Autodesk Inventor part; units mm, degrees
(part 2 of 2)
  spline S170 degree 2 poles (-5.6708, -24.2315) (-5.4763, -24.2315) (-5.2794, -24.0127) (-5.2794, -23.8036) knots 0 0 0 1 2 2 2
  spline S171 degree 2 poles (-5.2794, -23.8036) (-5.2794, -23.6261) (-5.4326, -23.3344) (-5.5468, -23.208) knots 0 0 0 1 2 2 2
  spline S172 degree 2 poles (-4.9925, -22.8773) (-4.9196, -22.9649) (-4.7032, -23.0961) (-4.6084, -23.0961) knots 0 0 0 1 2 2 2
  spline S173 degree 2 poles (-4.6084, -23.0961) (-4.5428, -23.0961) (-4.4601, -23.0208) (-4.4601, -22.9454) knots 0 0 0 1 2 2 2
  spline S174 degree 2 poles (-4.4601, -22.9454) (-4.4601, -22.9041) (-4.4796, -22.8287) (-4.4893, -22.8044) knots 0 0 0 1 2 2 2
  line L358 (-4.4893, -22.8044) -> (-4.4893, -22.7825)
  line L359 (-4.4893, -22.7825) -> (-4.2073, -22.7825)
  spline S175 degree 2 poles (-4.2073, -22.7825) (-4.183, -22.8409) (-4.1611, -22.9697) (-4.1611, -23.0232) knots 0 0 0 1 2 2 2
  spline S176 degree 2 poles (-4.1611, -23.0232) (-4.1611, -23.2031) (-4.3483, -23.4073) (-4.516, -23.4073) knots 0 0 0 1 2 2 2
  spline S177 degree 2 poles (-4.516, -23.4073) (-4.6473, -23.4073) (-4.9074, -23.2663) (-4.9925, -23.1764) knots 0 0 0 1 2 2 2
  line L360 (-4.9925, -23.1764) -> (-4.9925, -22.8773)
  spline S178 degree 2 poles (-4.9488, -21.6156) (-4.9488, -21.9243) (-5.3013, -22.272) (-5.683, -22.272) knots 0 0 0 1 2 2 2
  line L361 (-5.683, -22.272) -> (-6.9301, -22.272)
  line L362 (-6.9301, -22.272) -> (-6.9301, -22.5273)
  line L363 (-6.9301, -22.5273) -> (-7.2438, -22.5273)
  line L364 (-7.2438, -22.5273) -> (-7.2438, -22.272)
  line L365 (-7.2438, -22.272) -> (-7.8904, -22.272)
  line L366 (-7.8904, -22.272) -> (-7.8904, -21.8927)
  line L367 (-7.8904, -21.8927) -> (-7.2438, -21.8927)
  line L368 (-7.2438, -21.8927) -> (-7.2438, -21.195)
  line L369 (-7.2438, -21.195) -> (-6.9301, -21.195)
  line L370 (-6.9301, -21.195) -> (-6.9301, -21.8927)
  line L371 (-6.9301, -21.8927) -> (-5.858, -21.8927)
  spline S179 degree 2 poles (-5.858, -21.8927) (-5.6878, -21.8927) (-5.5006, -21.8806) (-5.4204, -21.8393) knots 0 0 0 1 2 2 2
  spline S180 degree 2 poles (-5.4204, -21.8393) (-5.3499, -21.8052) (-5.2794, -21.6521) (-5.2794, -21.5208) knots 0 0 0 1 2 2 2
  spline S181 degree 2 poles (-5.2794, -21.5208) (-5.2794, -21.4284) (-5.3353, -21.2558) (-5.3523, -21.2169) knots 0 0 0 1 2 2 2
  line L372 (-5.3523, -21.2169) -> (-5.3523, -21.195)
  line L373 (-5.3523, -21.195) -> (-5.012, -21.195)
  spline S182 degree 2 poles (-5.012, -21.195) (-4.9828, -21.302) (-4.9488, -21.5208) (-4.9488, -21.6156) knots 0 0 0 1 2 2 2
  line L374 (-7.2438, -19.148) -> (-4.1635, -20.3587)
  line L375 (-4.1635, -20.3587) -> (-4.1635, -20.7647)
  line L376 (-4.1635, -20.7647) -> (-5.1019, -20.3611)
  line L377 (-5.1019, -20.3611) -> (-7.2438, -21.178)
  line L378 (-7.2438, -21.178) -> (-7.2438, -20.7696)
  line L379 (-7.2438, -20.7696) -> (-5.576, -20.1545)
  line L380 (-5.576, -20.1545) -> (-7.2438, -19.5418)
  line L381 (-7.2438, -19.5418) -> (-7.2438, -19.148)
  line L382 (-5.1301, -41.1451) -> (-5.1301, -41.6022)
  line L383 (-5.1301, -41.6022) -> (-6.3262, -42.3315)
  line L384 (-6.3262, -42.3315) -> (-5.1301, -43.0754)
  line L385 (-5.1301, -43.0754) -> (-5.1301, -43.5057)
  line L386 (-5.1301, -43.5057) -> (-6.6325, -42.5503)
  line L387 (-6.6325, -42.5503) -> (-8.1301, -43.4765)
  line L388 (-8.1301, -43.4765) -> (-8.1301, -43.0195)
  line L389 (-8.1301, -43.0195) -> (-6.9558, -42.3047)
  line L390 (-6.9558, -42.3047) -> (-8.1301, -41.5754)
  line L391 (-8.1301, -41.5754) -> (-8.1301, -41.1451)
  line L392 (-8.1301, -41.1451) -> (-6.652, -42.0835)
  line L393 (-6.652, -42.0835) -> (-5.1301, -41.1451)
  line L394 (-8.1301, -38.7237) -> (-6.4575, -39.7375)
  line L395 (-6.4575, -39.7375) -> (-5.1301, -39.7375)
  line L396 (-5.1301, -39.7375) -> (-5.1301, -40.1362)
  line L397 (-5.1301, -40.1362) -> (-6.4161, -40.1362)
  line L398 (-6.4161, -40.1362) -> (-8.1301, -41.15)
  line L399 (-8.1301, -41.15) -> (-8.1301, -40.7075)
  line L400 (-8.1301, -40.7075) -> (-6.81, -39.9344)
  line L401 (-6.81, -39.9344) -> (-8.1301, -39.1467)
  line L402 (-8.1301, -39.1467) -> (-8.1301, -38.7237)
  line L403 (-5.1301, -36.5333) -> (-5.1301, -38.6289)
  line L404 (-5.1301, -38.6289) -> (-5.502, -38.6289)
  line L405 (-5.502, -38.6289) -> (-7.7751, -37.0244)
  line L406 (-7.7751, -37.0244) -> (-7.7751, -38.556)
  line L407 (-7.7751, -38.556) -> (-8.1301, -38.556)
  line L408 (-8.1301, -38.556) -> (-8.1301, -36.5746)
  line L409 (-8.1301, -36.5746) -> (-7.7703, -36.5746)
  line L410 (-7.7703, -36.5746) -> (-5.485, -38.1962)
  line L411 (-5.485, -38.1962) -> (-5.485, -36.5333)
  line L412 (-5.485, -36.5333) -> (-5.1301, -36.5333)
  spline S183 degree 2 poles (4.3705, -37.8576) (4.565, -37.8576) (4.9151, -37.9962) (5.0366, -38.1201) knots 0 0 0 1 2 2 2
  spline S184 degree 2 poles (5.0366, -38.1201) (5.1898, -38.2757) (5.3478, -38.6963) (5.3478, -39.0172) knots 0 0 0 1 2 2 2
  line L413 (5.3478, -39.0172) -> (5.3478, -39.3552)
  line L414 (5.3478, -39.3552) -> (6.4661, -39.3552)
  line L415 (6.4661, -39.3552) -> (6.4661, -39.7539)
  line L416 (6.4661, -39.7539) -> (3.4661, -39.7539)
  line L417 (3.4661, -39.7539) -> (3.4661, -39.0002)
  spline S185 degree 2 poles (3.4661, -39.0002) (3.4661, -38.7328) (3.5536, -38.3584) (3.6533, -38.215) knots 0 0 0 1 2 2 2
  spline S186 degree 2 poles (3.6533, -38.215) (3.7676, -38.0472) (4.1201, -37.8576) (4.3705, -37.8576) knots 0 0 0 1 2 2 2
  spline S187 degree 2 poles (4.3827, -38.2733) (4.2271, -38.2733) (3.9985, -38.3803) (3.9256, -38.4897) knots 0 0 0 1 2 2 2
  spline S188 degree 2 poles (3.9256, -38.4897) (3.8624, -38.5845) (3.8113, -38.8373) (3.8113, -39.0245) knots 0 0 0 1 2 2 2
  line L418 (3.8113, -39.0245) -> (3.8113, -39.3552)
  line L419 (3.8113, -39.3552) -> (5.0075, -39.3552)
  line L420 (5.0075, -39.3552) -> (5.0075, -39.0829)
  spline S189 degree 2 poles (5.0075, -39.0829) (5.0075, -38.8398) (4.9297, -38.5407) (4.8275, -38.4435) knots 0 0 0 1 2 2 2
  spline S190 degree 2 poles (4.8275, -38.4435) (4.7376, -38.3535) (4.5261, -38.2733) (4.3827, -38.2733) knots 0 0 0 1 2 2 2
  line L421 (4.6209, -36.3138) -> (4.6209, -36.3333)
  spline S191 degree 2 poles (4.6209, -36.3333) (4.6087, -36.377) (4.6039, -36.4719) (4.6039, -36.5375) knots 0 0 0 1 2 2 2
  spline S192 degree 2 poles (4.6039, -36.5375) (4.6039, -36.6907) (4.7376, -36.9921) (4.8689, -37.1283) knots 0 0 0 1 2 2 2
  line L422 (4.8689, -37.1283) -> (6.4661, -37.1283)
  line L423 (6.4661, -37.1283) -> (6.4661, -37.5075)
  line L424 (6.4661, -37.5075) -> (4.2149, -37.5075)
  line L425 (4.2149, -37.5075) -> (4.2149, -37.1283)
  line L426 (4.2149, -37.1283) -> (4.5504, -37.1283)
  spline S193 degree 2 poles (4.5504, -37.1283) (4.3656, -36.9216) (4.2149, -36.6129) (4.2149, -36.467) knots 0 0 0 1 2 2 2
  spline S194 degree 2 poles (4.2149, -36.467) (4.2149, -36.4086) (4.2198, -36.3503) (4.2271, -36.3138) knots 0 0 0 1 2 2 2
  line L427 (4.2271, -36.3138) -> (4.6209, -36.3138)
  line L428 (6.4661, -34.5415) -> (6.4661, -36.1947)
  line L429 (6.4661, -36.1947) -> (6.1841, -36.1947)
  line L430 (6.1841, -36.1947) -> (4.5261, -35.018)
  line L431 (4.5261, -35.018) -> (4.5261, -36.1461)
  line L432 (4.5261, -36.1461) -> (4.2149, -36.1461)
  line L433 (4.2149, -36.1461) -> (4.2149, -34.5634)
  line L434 (4.2149, -34.5634) -> (4.4848, -34.5634)
  line L435 (4.4848, -34.5634) -> (6.1476, -35.7449)
  line L436 (6.1476, -35.7449) -> (6.1476, -34.5415)
  line L437 (6.1476, -34.5415) -> (6.4661, -34.5415)
  spline S195 degree 2 poles (6.5172, -33.2093) (6.5172, -33.749) (5.9118, -34.3422) (5.3527, -34.3422) knots 0 0 0 1 2 2 2
  spline S196 degree 2 poles (5.3527, -34.3422) (4.8032, -34.3422) (4.1517, -33.766) (4.1517, -33.3017) knots 0 0 0 1 2 2 2
  spline S197 degree 2 poles (4.1517, -33.3017) (4.1517, -33.0926) (4.2733, -32.7693) (4.4021, -32.6501) knots 0 0 0 1 2 2 2
  spline S198 degree 2 poles (4.4021, -32.6501) (4.531, -32.5286) (4.9029, -32.3997) (5.1728, -32.3997) knots 0 0 0 1 2 2 2
  line L438 (5.1728, -32.3997) -> (5.3794, -32.3997)
  line L439 (5.3794, -32.3997) -> (5.3794, -33.9581)
  spline S199 degree 2 poles (5.3794, -33.9581) (5.7708, -33.9581) (6.1865, -33.5642) (6.1865, -33.2142) knots 0 0 0 1 2 2 2
  spline S200 degree 2 poles (6.1865, -33.2142) (6.1865, -33.0902) (6.1306, -32.8495) (6.0869, -32.7522) knots 0 0 0 1 2 2 2
  spline S201 degree 2 poles (6.0869, -32.7522) (6.0382, -32.6501) (5.9532, -32.5091) (5.9143, -32.4629) knots 0 0 0 1 2 2 2
  line L440 (5.9143, -32.4629) -> (5.9143, -32.4411)
  line L441 (5.9143, -32.4411) -> (6.3275, -32.4411)
  spline S202 degree 2 poles (6.3275, -32.4411) (6.3543, -32.5067) (6.4321, -32.706) (6.454, -32.7838) knots 0 0 0 1 2 2 2
  spline S203 degree 2 poles (6.454, -32.7838) (6.4856, -32.8932) (6.5172, -33.0731) (6.5172, -33.2093) knots 0 0 0 1 2 2 2
  spline S204 degree 2 poles (5.0901, -32.7693) (4.9369, -32.7741) (4.7133, -32.8373) (4.6379, -32.8981) knots 0 0 0 1 2 2 2
  spline S205 degree 2 poles (4.6379, -32.8981) (4.5528, -32.9637) (4.4629, -33.1704) (4.4629, -33.3236) knots 0 0 0 1 2 2 2
  spline S206 degree 2 poles (4.4629, -33.3236) (4.4629, -33.4743) (4.5528, -33.6858) (4.6404, -33.7733) knots 0 0 0 1 2 2 2
  spline S207 degree 2 poles (4.6404, -33.7733) (4.7303, -33.8584) (4.9467, -33.9459) (5.0901, -33.9581) knots 0 0 0 1 2 2 2
  line L442 (5.0901, -33.9581) -> (5.0901, -32.7693)
  spline S208 degree 2 poles (6.8259, -31.9354) (6.8429, -31.8965) (6.8964, -31.7482) (6.9183, -31.6534) knots 0 0 0 1 2 2 2
  spline S209 degree 2 poles (6.9183, -31.6534) (6.9451, -31.5488) (6.9767, -31.3714) (6.9767, -31.2668) knots 0 0 0 1 2 2 2
  spline S210 degree 2 poles (6.9767, -31.2668) (6.9767, -31.0918) (6.8843, -30.8487) (6.8016, -30.7806) knots 0 0 0 1 2 2 2
  spline S211 degree 2 poles (6.8016, -30.7806) (6.719, -30.715) (6.5026, -30.6639) (6.364, -30.6639) knots 0 0 0 1 2 2 2
  line L443 (6.364, -30.6639) -> (6.1671, -30.6639)
  spline S212 degree 2 poles (6.1671, -30.6639) (6.3008, -30.8171) (6.4272, -31.1112) (6.4272, -31.3325) knots 0 0 0 1 2 2 2
  spline S213 degree 2 poles (6.4272, -31.3325) (6.4272, -31.7166) (5.8559, -32.1712) (5.3186, -32.1712) knots 0 0 0 1 2 2 2
  spline S214 degree 2 poles (5.3186, -32.1712) (5.0391, -32.1712) (4.6063, -32.0132) (4.4532, -31.8819) knots 0 0 0 1 2 2 2
  spline S215 degree 2 poles (4.4532, -31.8819) (4.3097, -31.7555) (4.1517, -31.4078) (4.1517, -31.2231) knots 0 0 0 1 2 2 2
  spline S216 degree 2 poles (4.1517, -31.2231) (4.1517, -31.048) (4.2344, -30.7928) (4.3097, -30.6639) knots 0 0 0 1 2 2 2
  line L444 (4.3097, -30.6639) -> (4.2149, -30.642)
  line L445 (4.2149, -30.642) -> (4.2149, -30.2847)
  line L446 (4.2149, -30.2847) -> (6.2084, -30.2847)
  spline S217 degree 2 poles (6.2084, -30.2847) (6.7822, -30.2847) (7.317, -30.783) (7.317, -31.296) knots 0 0 0 1 2 2 2
  spline S218 degree 2 poles (7.317, -31.296) (7.317, -31.4613) (7.2635, -31.8065) (7.2198, -31.9548) knots 0 0 0 1 2 2 2
  line L447 (7.2198, -31.9548) -> (6.8259, -31.9548)
  line L448 (6.8259, -31.9548) -> (6.8259, -31.9354)
  line L449 (5.8559, -30.6639) -> (4.6185, -30.6639)
  spline S219 degree 2 poles (4.6185, -30.6639) (4.5504, -30.8049) (4.4921, -31.0432) (4.4921, -31.1623) knots 0 0 0 1 2 2 2
  spline S220 degree 2 poles (4.4921, -31.1623) (4.4921, -31.4492) (4.9151, -31.7798) (5.3113, -31.7798) knots 0 0 0 1 2 2 2
  spline S221 degree 2 poles (5.3113, -31.7798) (5.6857, -31.7798) (6.0771, -31.5294) (6.0771, -31.2474) knots 0 0 0 1 2 2 2
  spline S222 degree 2 poles (6.0771, -31.2474) (6.0771, -31.0991) (5.9605, -30.7879) (5.8559, -30.6639) knots 0 0 0 1 2 2 2
  line L450 (6.4661, -27.9848) -> (6.4661, -28.3641)
  line L451 (6.4661, -28.3641) -> (6.2181, -28.3641)
  spline S223 degree 2 poles (6.2181, -28.3641) (6.3713, -28.5391) (6.5293, -28.8527) (6.5293, -29.0472) knots 0 0 0 1 2 2 2
  spline S224 degree 2 poles (6.5293, -29.0472) (6.5293, -29.1931) (6.4321, -29.4532) (6.3275, -29.548) knots 0 0 0 1 2 2 2
  spline S225 degree 2 poles (6.3275, -29.548) (6.223, -29.6453) (5.9045, -29.7522) (5.676, -29.7522) knots 0 0 0 1 2 2 2
  line L452 (5.676, -29.7522) -> (4.2149, -29.7522)
  line L453 (4.2149, -29.7522) -> (4.2149, -29.373)
  line L454 (4.2149, -29.373) -> (5.4985, -29.373)
  spline S226 degree 2 poles (5.4985, -29.373) (5.6784, -29.373) (5.9143, -29.3462) (6.0018, -29.3001) knots 0 0 0 1 2 2 2
  spline S227 degree 2 poles (6.0018, -29.3001) (6.0893, -29.2539) (6.1695, -29.0958) (6.1695, -28.9475) knots 0 0 0 1 2 2 2
  spline S228 degree 2 poles (6.1695, -28.9475) (6.1695, -28.809) (6.0115, -28.4954) (5.8972, -28.3641) knots 0 0 0 1 2 2 2
  line L455 (5.8972, -28.3641) -> (4.2149, -28.3641)
  line L456 (4.2149, -28.3641) -> (4.2149, -27.9848)
  line L457 (4.2149, -27.9848) -> (6.4661, -27.9848)
  spline S229 degree 2 poles (5.304, -25.5488) (5.8559, -25.5488) (6.5293, -26.0837) (6.5293, -26.4872) knots 0 0 0 1 2 2 2
  spline S230 degree 2 poles (6.5293, -26.4872) (6.5293, -26.6696) (6.4394, -26.9297) (6.3616, -27.0561) knots 0 0 0 1 2 2 2
  line L458 (6.3616, -27.0561) -> (6.4661, -27.0804)
  line L459 (6.4661, -27.0804) -> (6.4661, -27.4354)
  line L460 (6.4661, -27.4354) -> (3.3324, -27.4354)
  line L461 (3.3324, -27.4354) -> (3.3324, -27.0561)
  line L462 (3.3324, -27.0561) -> (4.4507, -27.0561)
  spline S231 degree 2 poles (4.4507, -27.0561) (4.3219, -26.9127) (4.1517, -26.5796) (4.1517, -26.3681) knots 0 0 0 1 2 2 2
  spline S232 degree 2 poles (4.1517, -26.3681) (4.1517, -25.9864) (4.7619, -25.5488) (5.304, -25.5488) knots 0 0 0 1 2 2 2
  spline S233 degree 2 poles (5.3332, -25.9402) (4.9297, -25.9402) (4.5115, -26.1858) (4.5115, -26.4581) knots 0 0 0 1 2 2 2
  spline S234 degree 2 poles (4.5115, -26.4581) (4.5115, -26.6112) (4.6574, -26.9273) (4.7692, -27.0561) knots 0 0 0 1 2 2 2
  line L463 (4.7692, -27.0561) -> (6.0601, -27.0561)
  spline S235 degree 2 poles (6.0601, -27.0561) (6.1306, -26.9127) (6.189, -26.6915) (6.189, -26.5602) knots 0 0 0 1 2 2 2
  spline S236 degree 2 poles (6.189, -26.5602) (6.189, -26.2709) (5.7781, -25.9402) (5.3332, -25.9402) knots 0 0 0 1 2 2 2
  line L464 (4.2149, -23.3876) -> (7.2951, -24.5983)
  line L465 (7.2951, -24.5983) -> (7.2951, -25.0043)
  line L466 (7.2951, -25.0043) -> (6.3567, -24.6007)
  line L467 (6.3567, -24.6007) -> (4.2149, -25.4176)
  line L468 (4.2149, -25.4176) -> (4.2149, -25.0091)
  line L469 (4.2149, -25.0091) -> (5.8827, -24.3941)
  line L470 (5.8827, -24.3941) -> (4.2149, -23.7814)
  line L471 (4.2149, -23.7814) -> (4.2149, -23.3876)
  line L472 (-14.143, -43.1956) -> (-16.7881, -43.1956)
  line L473 (-16.7881, -43.1956) -> (-16.7881, -44.2021)
  line L474 (-16.7881, -44.2021) -> (-17.143, -44.2021)
  line L475 (-17.143, -44.2021) -> (-17.143, -41.7904)
  line L476 (-17.143, -41.7904) -> (-16.7881, -41.7904)
  line L477 (-16.7881, -41.7904) -> (-16.7881, -42.7969)
  line L478 (-16.7881, -42.7969) -> (-14.143, -42.7969)
  line L479 (-14.143, -42.7969) -> (-14.143, -43.1956)
  line L480 (-15.9883, -40.322) -> (-15.9883, -40.3415)
  spline S237 degree 2 poles (-15.9883, -40.3415) (-16.0004, -40.3853) (-16.0053, -40.4801) (-16.0053, -40.5457) knots 0 0 0 1 2 2 2
  spline S238 degree 2 poles (-16.0053, -40.5457) (-16.0053, -40.6989) (-15.8716, -41.0003) (-15.7403, -41.1365) knots 0 0 0 1 2 2 2
  line L481 (-15.7403, -41.1365) -> (-14.143, -41.1365)
  line L482 (-14.143, -41.1365) -> (-14.143, -41.5157)
  line L483 (-14.143, -41.5157) -> (-16.3943, -41.5157)
  line L484 (-16.3943, -41.5157) -> (-16.3943, -41.1365)
  line L485 (-16.3943, -41.1365) -> (-16.0588, -41.1365)
  spline S239 degree 2 poles (-16.0588, -41.1365) (-16.2435, -40.9298) (-16.3943, -40.6211) (-16.3943, -40.4752) knots 0 0 0 1 2 2 2
  spline S240 degree 2 poles (-16.3943, -40.4752) (-16.3943, -40.4169) (-16.3894, -40.3585) (-16.3821, -40.322) knots 0 0 0 1 2 2 2
  line L486 (-16.3821, -40.322) -> (-15.9883, -40.322)
  line L487 (-16.3943, -38.2605) -> (-13.314, -39.4712)
  line L488 (-13.314, -39.4712) -> (-13.314, -39.8772)
  line L489 (-13.314, -39.8772) -> (-14.2524, -39.4736)
  line L490 (-14.2524, -39.4736) -> (-16.3943, -40.2904)
  line L491 (-16.3943, -40.2904) -> (-16.3943, -39.882)
  line L492 (-16.3943, -39.882) -> (-14.7265, -39.2669)
  line L493 (-14.7265, -39.2669) -> (-16.3943, -38.6543)
  line L494 (-16.3943, -38.6543) -> (-16.3943, -38.2605)
  spline S241 degree 2 poles (-15.3051, -36.087) (-14.7532, -36.087) (-14.0798, -36.6219) (-14.0798, -37.0254) knots 0 0 0 1 2 2 2
  spline S242 degree 2 poles (-14.0798, -37.0254) (-14.0798, -37.2078) (-14.1698, -37.4679) (-14.2476, -37.5943) knots 0 0 0 1 2 2 2
  line L495 (-14.2476, -37.5943) -> (-14.143, -37.6186)
  line L496 (-14.143, -37.6186) -> (-14.143, -37.9736)
  line L497 (-14.143, -37.9736) -> (-17.2767, -37.9736)
  line L498 (-17.2767, -37.9736) -> (-17.2767, -37.5943)
  line L499 (-17.2767, -37.5943) -> (-16.1584, -37.5943)
  spline S243 degree 2 poles (-16.1584, -37.5943) (-16.2873, -37.4509) (-16.4575, -37.1178) (-16.4575, -36.9063) knots 0 0 0 1 2 2 2
  spline S244 degree 2 poles (-16.4575, -36.9063) (-16.4575, -36.5246) (-15.8473, -36.087) (-15.3051, -36.087) knots 0 0 0 1 2 2 2
  spline S245 degree 2 poles (-15.2759, -36.4784) (-15.6795, -36.4784) (-16.0977, -36.724) (-16.0977, -36.9963) knots 0 0 0 1 2 2 2
  spline S246 degree 2 poles (-16.0977, -36.9963) (-16.0977, -37.1494) (-15.9518, -37.4655) (-15.84, -37.5943) knots 0 0 0 1 2 2 2
  line L500 (-15.84, -37.5943) -> (-14.549, -37.5943)
  spline S247 degree 2 poles (-14.549, -37.5943) (-14.4785, -37.4509) (-14.4202, -37.2297) (-14.4202, -37.0984) knots 0 0 0 1 2 2 2
  spline S248 degree 2 poles (-14.4202, -37.0984) (-14.4202, -36.8091) (-14.831, -36.4784) (-15.2759, -36.4784) knots 0 0 0 1 2 2 2
  spline S249 degree 2 poles (-14.0896, -33.5392) (-14.0896, -33.865) (-14.2257, -34.322) (-14.3229, -34.5238) knots 0 0 0 1 2 2 2
  line L501 (-14.3229, -34.5238) -> (-14.8237, -34.5238)
  line L502 (-14.8237, -34.5238) -> (-14.8237, -34.4947)
  spline S250 degree 2 poles (-14.8237, -34.4947) (-14.639, -34.2977) (-14.4348, -33.7994) (-14.4348, -33.5684) knots 0 0 0 1 2 2 2
  spline S251 degree 2 poles (-14.4348, -33.5684) (-14.4348, -33.2378) (-14.7095, -32.8998) (-14.9356, -32.8998) knots 0 0 0 1 2 2 2
  spline S252 degree 2 poles (-14.9356, -32.8998) (-15.1155, -32.8998) (-15.3391, -33.0773) (-15.3951, -33.2694) knots 0 0 0 1 2 2 2
  spline S253 degree 2 poles (-15.3951, -33.2694) (-15.434, -33.4079) (-15.4874, -33.6389) (-15.5312, -33.8115) knots 0 0 0 1 2 2 2
  spline S254 degree 2 poles (-15.5312, -33.8115) (-15.5725, -33.9671) (-15.6965, -34.2126) (-15.7962, -34.3075) knots 0 0 0 1 2 2 2
  spline S255 degree 2 poles (-15.7962, -34.3075) (-15.8959, -34.3998) (-16.1633, -34.5019) (-16.3383, -34.5019) knots 0 0 0 1 2 2 2
  spline S256 degree 2 poles (-16.3383, -34.5019) (-16.703, -34.5019) (-17.1965, -33.9331) (-17.1965, -33.493) knots 0 0 0 1 2 2 2
  spline S257 degree 2 poles (-17.1965, -33.493) (-17.1965, -33.2402) (-17.0968, -32.7929) (-17.002, -32.6008) knots 0 0 0 1 2 2 2
  line L503 (-17.002, -32.6008) -> (-16.5255, -32.6008)
  line L504 (-16.5255, -32.6008) -> (-16.5255, -32.63)
  spline S258 degree 2 poles (-16.5255, -32.63) (-16.6568, -32.7734) (-16.8513, -33.2207) (-16.8513, -33.4663) knots 0 0 0 1 2 2 2
  spline S259 degree 2 poles (-16.8513, -33.4663) (-16.8513, -33.7434) (-16.5912, -34.0862) (-16.3797, -34.0862) knots 0 0 0 1 2 2 2
  spline S260 degree 2 poles (-16.3797, -34.0862) (-16.19, -34.0862) (-15.9639, -33.8844) (-15.9129, -33.6948) knots 0 0 0 1 2 2 2
  spline S261 degree 2 poles (-15.9129, -33.6948) (-15.8789, -33.5684) (-15.7913, -33.2013) (-15.7549, -33.0797) knots 0 0 0 1 2 2 2
  spline S262 degree 2 poles (-15.7549, -33.0797) (-15.6601, -32.771) (-15.2784, -32.4841) (-14.9988, -32.4841) knots 0 0 0 1 2 2 2
  spline S263 degree 2 poles (-14.9988, -32.4841) (-14.8213, -32.4841) (-14.481, -32.6276) (-14.3618, -32.7564) knots 0 0 0 1 2 2 2
  spline S264 degree 2 poles (-14.3618, -32.7564) (-14.2306, -32.8998) (-14.0896, -33.2645) (-14.0896, -33.5392) knots 0 0 0 1 2 2 2
  spline S265 degree 2 poles (-14.0993, -31.4266) (-14.0993, -31.7353) (-14.4518, -32.083) (-14.8335, -32.083) knots 0 0 0 1 2 2 2
  line L505 (-14.8335, -32.083) -> (-16.0806, -32.083)
  line L506 (-16.0806, -32.083) -> (-16.0806, -32.3383)
  line L507 (-16.0806, -32.3383) -> (-16.3943, -32.3383)
  line L508 (-16.3943, -32.3383) -> (-16.3943, -32.083)
  line L509 (-16.3943, -32.083) -> (-17.0409, -32.083)
  line L510 (-17.0409, -32.083) -> (-17.0409, -31.7037)
  line L511 (-17.0409, -31.7037) -> (-16.3943, -31.7037)
  line L512 (-16.3943, -31.7037) -> (-16.3943, -31.006)
  line L513 (-16.3943, -31.006) -> (-16.0806, -31.006)
  line L514 (-16.0806, -31.006) -> (-16.0806, -31.7037)
  line L515 (-16.0806, -31.7037) -> (-15.0085, -31.7037)
  spline S266 degree 2 poles (-15.0085, -31.7037) (-14.8383, -31.7037) (-14.6511, -31.6916) (-14.5709, -31.6502) knots 0 0 0 1 2 2 2
  spline S267 degree 2 poles (-14.5709, -31.6502) (-14.5004, -31.6162) (-14.4299, -31.4631) (-14.4299, -31.3318) knots 0 0 0 1 2 2 2
  spline S268 degree 2 poles (-14.4299, -31.3318) (-14.4299, -31.2394) (-14.4858, -31.0668) (-14.5028, -31.0279) knots 0 0 0 1 2 2 2
  line L516 (-14.5028, -31.0279) -> (-14.5028, -31.006)
  line L517 (-14.5028, -31.006) -> (-14.1625, -31.006)
  spline S269 degree 2 poles (-14.1625, -31.006) (-14.1333, -31.113) (-14.0993, -31.3318) (-14.0993, -31.4266) knots 0 0 0 1 2 2 2
  spline S270 degree 2 poles (-14.092, -29.7491) (-14.092, -30.2888) (-14.6973, -30.882) (-15.2565, -30.882) knots 0 0 0 1 2 2 2
  spline S271 degree 2 poles (-15.2565, -30.882) (-15.8059, -30.882) (-16.4575, -30.3058) (-16.4575, -29.8415) knots 0 0 0 1 2 2 2
  spline S272 degree 2 poles (-16.4575, -29.8415) (-16.4575, -29.6324) (-16.3359, -29.3091) (-16.2071, -29.19) knots 0 0 0 1 2 2 2
  spline S273 degree 2 poles (-16.2071, -29.19) (-16.0782, -29.0684) (-15.7062, -28.9395) (-15.4364, -28.9395) knots 0 0 0 1 2 2 2
  line L518 (-15.4364, -28.9395) -> (-15.2297, -28.9395)
  line L519 (-15.2297, -28.9395) -> (-15.2297, -30.4979)
  spline S274 degree 2 poles (-15.2297, -30.4979) (-14.8383, -30.4979) (-14.4226, -30.1041) (-14.4226, -29.754) knots 0 0 0 1 2 2 2
  spline S275 degree 2 poles (-14.4226, -29.754) (-14.4226, -29.63) (-14.4785, -29.3893) (-14.5223, -29.2921) knots 0 0 0 1 2 2 2
  spline S276 degree 2 poles (-14.5223, -29.2921) (-14.5709, -29.19) (-14.656, -29.0489) (-14.6949, -29.0028) knots 0 0 0 1 2 2 2
  line L520 (-14.6949, -29.0028) -> (-14.6949, -28.9809)
  line L521 (-14.6949, -28.9809) -> (-14.2816, -28.9809)
  spline S277 degree 2 poles (-14.2816, -28.9809) (-14.2549, -29.0465) (-14.1771, -29.2459) (-14.1552, -29.3237) knots 0 0 0 1 2 2 2
  spline S278 degree 2 poles (-14.1552, -29.3237) (-14.1236, -29.4331) (-14.092, -29.613) (-14.092, -29.7491) knots 0 0 0 1 2 2 2
  spline S279 degree 2 poles (-15.519, -29.3091) (-15.6722, -29.3139) (-15.8959, -29.3772) (-15.9712, -29.4379) knots 0 0 0 1 2 2 2
  spline S280 degree 2 poles (-15.9712, -29.4379) (-16.0563, -29.5036) (-16.1463, -29.7102) (-16.1463, -29.8634) knots 0 0 0 1 2 2 2
  spline S281 degree 2 poles (-16.1463, -29.8634) (-16.1463, -30.0141) (-16.0563, -30.2256) (-15.9688, -30.3131) knots 0 0 0 1 2 2 2
  spline S282 degree 2 poles (-15.9688, -30.3131) (-15.8789, -30.3982) (-15.6625, -30.4857) (-15.519, -30.4979) knots 0 0 0 1 2 2 2
  line L522 (-15.519, -30.4979) -> (-15.519, -29.3091)
  line L523 (-15.9883, -27.3618) -> (-15.9883, -27.3812)
  spline S283 degree 2 poles (-15.9883, -27.3812) (-16.0004, -27.425) (-16.0053, -27.5198) (-16.0053, -27.5854) knots 0 0 0 1 2 2 2
  spline S284 degree 2 poles (-16.0053, -27.5854) (-16.0053, -27.7386) (-15.8716, -28.04) (-15.7403, -28.1762) knots 0 0 0 1 2 2 2
  line L524 (-15.7403, -28.1762) -> (-14.143, -28.1762)
  line L525 (-14.143, -28.1762) -> (-14.143, -28.5554)
  line L526 (-14.143, -28.5554) -> (-16.3943, -28.5554)
  line L527 (-16.3943, -28.5554) -> (-16.3943, -28.1762)
  line L528 (-16.3943, -28.1762) -> (-16.0588, -28.1762)
  spline S285 degree 2 poles (-16.0588, -28.1762) (-16.2435, -27.9695) (-16.3943, -27.6608) (-16.3943, -27.5149) knots 0 0 0 1 2 2 2
  spline S286 degree 2 poles (-16.3943, -27.5149) (-16.3943, -27.4566) (-16.3894, -27.3982) (-16.3821, -27.3618) knots 0 0 0 1 2 2 2
  line L529 (-16.3821, -27.3618) -> (-15.9883, -27.3618)
  spline S287 degree 2 poles (-15.2686, -25.2175) (-14.6998, -25.2175) (-14.0798, -25.7645) (-14.0798, -26.2216) knots 0 0 0 1 2 2 2
  spline S288 degree 2 poles (-14.0798, -26.2216) (-14.0798, -26.6908) (-14.7192, -27.228) (-15.2686, -27.228) knots 0 0 0 1 2 2 2
  spline S289 degree 2 poles (-15.2686, -27.228) (-15.8327, -27.228) (-16.4575, -26.6737) (-16.4575, -26.2216) knots 0 0 0 1 2 2 2
  spline S290 degree 2 poles (-16.4575, -26.2216) (-16.4575, -25.7645) (-15.8351, -25.2175) (-15.2686, -25.2175) knots 0 0 0 1 2 2 2
  spline S291 degree 2 poles (-15.2686, -25.6089) (-15.7062, -25.6089) (-16.1317, -25.9274) (-16.1317, -26.2216) knots 0 0 0 1 2 2 2
  spline S292 degree 2 poles (-16.1317, -26.2216) (-16.1317, -26.5157) (-15.7062, -26.8366) (-15.2686, -26.8366) knots 0 0 0 1 2 2 2
  spline S293 degree 2 poles (-15.2686, -26.8366) (-14.8432, -26.8366) (-14.4056, -26.5157) (-14.4056, -26.2216) knots 0 0 0 1 2 2 2
  spline S294 degree 2 poles (-14.4056, -26.2216) (-14.4056, -25.9298) (-14.8359, -25.6089) (-15.2686, -25.6089) knots 0 0 0 1 2 2 2
  line L530 (-16.3943, -22.1008) -> (-14.143, -22.6721)
  line L531 (-14.143, -22.6721) -> (-14.143, -23.0222)
  line L532 (-14.143, -23.0222) -> (-15.8789, -23.5716)
  line L533 (-15.8789, -23.5716) -> (-14.143, -24.1186)
  line L534 (-14.143, -24.1186) -> (-14.143, -24.4663)
  line L535 (-14.143, -24.4663) -> (-16.3943, -25.0425)
  line L536 (-16.3943, -25.0425) -> (-16.3943, -24.6486)
  line L537 (-16.3943, -24.6486) -> (-14.6511, -24.2499)
  line L538 (-14.6511, -24.2499) -> (-16.3943, -23.7175)
  line L539 (-16.3943, -23.7175) -> (-16.3943, -23.4039)
  line L540 (-16.3943, -23.4039) -> (-14.6511, -22.8569)
  line L541 (-14.6511, -22.8569) -> (-16.3943, -22.4825)
  line L542 (-16.3943, -22.4825) -> (-16.3943, -22.1008)
  line L543 (-14.143, -20.0003) -> (-14.143, -20.3796)
  line L544 (-14.143, -20.3796) -> (-15.4267, -20.3796)
  spline S295 degree 2 poles (-15.4267, -20.3796) (-15.5823, -20.3796) (-15.8497, -20.4088) (-15.9299, -20.4525) knots 0 0 0 1 2 2 2
  spline S296 degree 2 poles (-15.9299, -20.4525) (-16.015, -20.4987) (-16.0977, -20.664) (-16.0977, -20.805) knots 0 0 0 1 2 2 2
  spline S297 degree 2 poles (-16.0977, -20.805) (-16.0977, -20.946) (-15.9469, -21.2451) (-15.8254, -21.3885) knots 0 0 0 1 2 2 2
  line L545 (-15.8254, -21.3885) -> (-14.143, -21.3885)
  line L546 (-14.143, -21.3885) -> (-14.143, -21.7678)
  line L547 (-14.143, -21.7678) -> (-16.3943, -21.7678)
  line L548 (-16.3943, -21.7678) -> (-16.3943, -21.3885)
  line L549 (-16.3943, -21.3885) -> (-16.1438, -21.3885)
  spline S298 degree 2 poles (-16.1438, -21.3885) (-16.297, -21.2183) (-16.4575, -20.8901) (-16.4575, -20.7054) knots 0 0 0 1 2 2 2
  spline S299 degree 2 poles (-16.4575, -20.7054) (-16.4575, -20.3747) (-16.0199, -20.0003) (-15.6041, -20.0003) knots 0 0 0 1 2 2 2
  line L550 (-15.6041, -20.0003) -> (-14.143, -20.0003)
  line L551 (-14.143, -19.0814) -> (-14.143, -19.4606)
  line L552 (-14.143, -19.4606) -> (-16.3943, -19.4606)
  line L553 (-16.3943, -19.4606) -> (-16.3943, -19.0814)
  line L554 (-16.3943, -19.0814) -> (-14.143, -19.0814)
  line L555 (-16.7686, -19.0546) -> (-16.7686, -19.4849)
  line L556 (-16.7686, -19.4849) -> (-17.1625, -19.4849)
  line L557 (-17.1625, -19.4849) -> (-17.1625, -19.0546)
  line L558 (-17.1625, -19.0546) -> (-16.7686, -19.0546)
  spline S300 degree 2 poles (-14.3813, -17.2702) (-14.3473, -17.3164) (-14.2257, -17.472) (-14.1892, -17.5449) knots 0 0 0 1 2 2 2
  spline S301 degree 2 poles (-14.1892, -17.5449) (-14.1357, -17.6446) (-14.0798, -17.8318) (-14.0798, -18.0019) knots 0 0 0 1 2 2 2
  spline S302 degree 2 poles (-14.0798, -18.0019) (-14.0798, -18.1405) (-14.1844, -18.3909) (-14.2792, -18.4857) knots 0 0 0 1 2 2 2
  spline S303 degree 2 poles (-14.2792, -18.4857) (-14.3716, -18.5757) (-14.6438, -18.6851) (-14.7946, -18.6851) knots 0 0 0 1 2 2 2
  spline S304 degree 2 poles (-14.7946, -18.6851) (-15.028, -18.6851) (-15.3586, -18.4882) (-15.4534, -18.2742) knots 0 0 0 1 2 2 2
  spline S305 degree 2 poles (-15.4534, -18.2742) (-15.5409, -18.0846) (-15.6066, -17.5692) (-15.6236, -17.2702) knots 0 0 0 1 2 2 2
  line L559 (-15.6236, -17.2702) -> (-15.6965, -17.2702)
  spline S306 degree 2 poles (-15.6965, -17.2702) (-15.8278, -17.2702) (-15.9907, -17.3504) (-16.0369, -17.4233) knots 0 0 0 1 2 2 2
  spline S307 degree 2 poles (-16.0369, -17.4233) (-16.0831, -17.4963) (-16.1122, -17.7054) (-16.1122, -17.8172) knots 0 0 0 1 2 2 2
  spline S308 degree 2 poles (-16.1122, -17.8172) (-16.1122, -17.9485) (-16.0344, -18.3034) (-15.9591, -18.4809) knots 0 0 0 1 2 2 2
  line L560 (-15.9591, -18.4809) -> (-15.9591, -18.5028)
  line L561 (-15.9591, -18.5028) -> (-16.3456, -18.5028)
  spline S309 degree 2 poles (-16.3456, -18.5028) (-16.3748, -18.3982) (-16.4477, -18.0068) (-16.4477, -17.8148) knots 0 0 0 1 2 2 2
  spline S310 degree 2 poles (-16.4477, -17.8148) (-16.4477, -17.5814) (-16.3748, -17.2629) (-16.28, -17.1365) knots 0 0 0 1 2 2 2
  spline S311 degree 2 poles (-16.28, -17.1365) (-16.1876, -17.0125) (-15.8934, -16.8909) (-15.6819, -16.8909) knots 0 0 0 1 2 2 2
  line L562 (-15.6819, -16.8909) -> (-14.143, -16.8909)
  line L563 (-14.143, -16.8909) -> (-14.143, -17.2702)
  line L564 (-14.143, -17.2702) -> (-14.3813, -17.2702)
  line L565 (-14.6973, -17.2702) -> (-15.3221, -17.2702)
  spline S312 degree 2 poles (-15.3221, -17.2702) (-15.31, -17.4063) (-15.2686, -17.8172) (-15.2297, -17.946) knots 0 0 0 1 2 2 2
  spline S313 degree 2 poles (-15.2297, -17.946) (-15.1836, -18.0968) (-14.9915, -18.2937) (-14.8213, -18.2937) knots 0 0 0 1 2 2 2
  spline S314 degree 2 poles (-14.8213, -18.2937) (-14.6268, -18.2937) (-14.4299, -18.0749) (-14.4299, -17.8658) knots 0 0 0 1 2 2 2
  spline S315 degree 2 poles (-14.4299, -17.8658) (-14.4299, -17.6883) (-14.5831, -17.3966) (-14.6973, -17.2702) knots 0 0 0 1 2 2 2
  point P0 (0, 0)
  constraints: 4 end point, 2 horizontal, 1 point on line, 26 other
extrude "Wyciągnięcie proste3" cut sketch "Szkic4" against normal blind 0.2
sketch "Szkic5" plane through (0, 5, 0) normal (0, 1, 0) x (1, 0, 0)
  line L0 (-27.5, 50) -> (-27.5, -50) projected
  line L1 (-27.5, 0) -> (-22.5, 0)
  line L2 (27.5, -50) -> (27.5, 50) projected
  line L3 (27.5, 0) -> (22.5, 0)
  circle A0 centre (22.5, 0) radius 2.75
  circle A1 centre (-22.5, 0) radius 2.75
  circle A2 centre (-22.5, 0) radius 4.5
  circle A3 centre (22.5, 0) radius 4.5
  point P0 (0, 0)
  dimension "d56" = 5
  dimension "d57" = 5
  dimension "d58" = 5.5
  dimension "d59" = 5.5
  dimension "d60" = 9
  dimension "d61" = 9
  constraints: 4 centre point, 4 coincident, 4 end point, 2 horizontal, 2 midpoint
  measures "d56" distance of L1.start L1.end
  measures "d57" distance of L3.start L3.end
  measures "d58" diameter of A0
  measures "d59" diameter of A1
  measures "d60" diameter of A2
  measures "d61" diameter of A3
extrude "Wyciągnięcie proste4" add sketch "Szkic5" against normal blind 23
fillet "Zaokrąglenie1" radius 9 4 edges at (-27.5, 2.5, 50) (-27.5, 2.5, -50) (27.5, 2.5, -50) (27.5, 2.5, 50)
